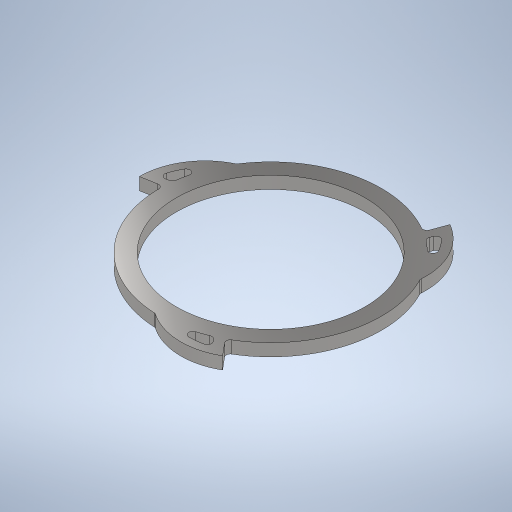
# Autodesk Inventor part: Blade V2
Saved by Autodesk Inventor 2023.2 (Build 272271000, 271)
## iProperties
Created: 2022-12-02
Part Number: Blade V2
Material: Stainless Steel
Document SubType Name: Modeling
Designer: Nathan Cai
Density: 8 g/cm^3
Appearance: Semi-Polished
Mass: 578.498 g
Surface Area: 266.036 cm^2
Volume: 72.3123 cm^3
Ring_ID: 5.750 in
ToothDepth: 0.625 in
RingWD: 0.500 in
Author: Nathan Cai
Autodesk Inventor part; units mm, degrees
ref_plane "YZ Plane" through (0, 0, 0) normal (1, 0, 0) x (0, 1, 0)
ref_plane "XZ Plane" through (0, 0, 0) normal (0, 1, 0) x (-1, 0, 0)
ref_plane "XY Plane" through (0, 0, 0) normal (0, 0, 1) x (1, 0, 0)
sketch "Sketch1" plane through (0, 0, 0) normal (0, 1, 0) x (-1, 0, 0)
  circle A0 centre (0, 0) radius 73.025
  circle A1 centre (0, 0) radius 85.725
  line L0 (0, 0) -> (101.6, 0) construction
  line L1 (101.6, 0) -> (85.679, -2.8073)
  arc A2 (72.3305, -46.0117) -> (101.6, 0) centre (50.8, 0) ccw
  line L2 (-50.8, 87.9882) -> (-40.4083, 75.6039)
  arc A3 (3.6821, 85.6459) -> (-50.8, 87.9882) centre (-25.4, 43.9941) ccw
  line L3 (-50.8, -87.9882) -> (-45.2707, -72.7966)
  arc A4 (-76.0126, -39.6342) -> (-50.8, -87.9882) centre (-25.4, -43.9941) ccw
  arc A5 (78.2836, -34.935) -> (94.5805, -7.6857) centre (50.8, 0) ccw
  line L4 (94.5805, -7.6857) -> (85.215, -9.3371)
  line L5 (-40.6343, 85.752) -> (-34.5213, 78.4669)
  arc A6 (-8.8872, 85.2631) -> (-40.6343, 85.752) centre (-25.4, 43.9941) ccw
  line L6 (-53.9463, -78.0663) -> (-50.6936, -69.1298)
  arc A7 (-69.3964, -50.3281) -> (-53.9463, -78.0663) centre (-25.4, -43.9941) ccw
  point P0 (85.725, 0)
  point P1 (-42.8625, 74.24)
  point P2 (-42.8625, -74.24)
  point P3 (-8.8872, 85.2631)
  dimension "Ring_ID" = 146.05
  dimension "RingWD" = 12.7
  dimension "ToothDepth" = 15.875
  dimension "d4" = 10
  dimension "d5" = 50.8
  dimension "d8" = 360
  dimension "d13" = 6.35
  dimension "d14" = 6.35
  dimension "d17" = 360
  constraints: 17 point on circle, 14 end point, 8 centre point, 2 coincident, 1 horizontal, 1 line through centre, 1 point on line, 41 other
  measures "Ring_ID" diameter of A0
  measures "RingWD" radial gap between concentric circles of A1 A0
  measures "ToothDepth" distance of A1.start L0.end
  measures "d4" angle of L0 L1
  measures "d5" radius of A2
  measures "d13" radial gap between concentric circles of A2 A5
  measures "d14" distance between parallel lines of L1 L4
extrude "Extrusion1" add sketch "Sketch1" along normal blind 9.525 contours A1 | A1 A6 L5 L2 A3 | L1 A2 A1 A5 L4 | A1 A7 L6 L3 A4
fillet "Fillet1" radius 3.175 6 edges at (40.4083, 4.7625, 75.6039) (-3.6821, 4.7625, 85.6459) (76.0126, 4.7625, -39.6342) (45.2707, 4.7625, -72.7966) (-85.679, 4.7625, -2.8073) (-72.3305, 4.7625, -46.0117)
fillet "Fillet2" radius 3.175 9 edges at (53.9463, 4.7625, -78.0663) (50.6936, 4.7625, -69.1298) (69.3964, 4.7625, -50.3281) (-94.5805, 4.7625, -7.6857) (-85.215, 4.7625, -9.3371) (-78.2836, 4.7625, -34.935) (40.6343, 4.7625, 85.752) (34.5213, 4.7625, 78.4669) (8.8872, 4.7625, 85.2631)
body "Solid1"
